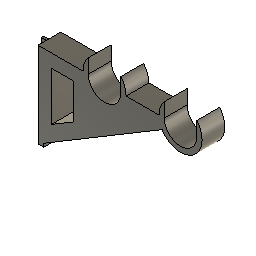
spool_cradle_bracket (Autodesk Fusion 360 design; units mm, degrees)
part number: 2026-09-02-15-42-23-246
Autodesk Fusion 360 part; units mm, degrees
sketch "Arm triangle" plane through (0, 0, 0) normal (0, 1, 0) x (1, 0, 0)
  line L0 (0, 0) -> (0, -90)
  line L1 (0, -90) -> (150, -90)
  line L2 (150, -90) -> (0, 0)
extrude "Arm triangle (1)" add sketch "Arm triangle" along normal mid plane 24
sketch "Hook plate" plane through (0, 0, 0) normal (0, 1, 0) x (1, 0, 0)
  line L0 (0, 0) -> (6, 0)
  line L1 (6, 0) -> (6, -90)
  line L2 (6, -90) -> (0, -90)
  line L3 (0, -90) -> (0, 0)
extrude "Hook plate (1)" add sketch "Hook plate" along normal mid plane 24
sketch "Lightening cutout" plane through (0, 0, 0) normal (0, 1, 0) x (1, 0, 0)
  line L0 (14, -24.7267) -> (14, -76)
  line L1 (14, -76) -> (37.3, -76)
  line L2 (37.3, -76) -> (37.3, -38.7067)
  line L3 (37.3, -38.7067) -> (14, -24.7267)
extrude "Lightening cutout (1)" cut sketch "Lightening cutout" along normal mid plane 34
sketch "Saddle boss x=70" plane through (0, 0, 0) normal (0, 1, 0) x (1, 0, 0)
  circle A0 centre (70, -90) radius 22.7
extrude "Saddle boss x=70 (1)" add sketch "Saddle boss x=70" along normal mid plane 24
sketch "Saddle boss x=150" plane through (0, 0, 0) normal (0, 1, 0) x (1, 0, 0)
  circle A0 centre (150, -90) radius 22.7
extrude "Saddle boss x=150 (1)" add sketch "Saddle boss x=150" along normal mid plane 24
sketch "Rod pocket x=70" plane through (0, 0, 0) normal (0, 1, 0) x (1, 0, 0)
  circle A0 centre (70, -90) radius 17.1
extrude "Rod pocket x=70 (1)" cut sketch "Rod pocket x=70" along normal mid plane 34
sketch "Drop-in opening x=70" plane through (0, 0, 0) normal (0, 1, 0) x (1, 0, 0)
  line L0 (52.9, -90) -> (87.1, -90)
  line L1 (87.1, -90) -> (87.1, -117.7)
  line L2 (87.1, -117.7) -> (52.9, -117.7)
  line L3 (52.9, -117.7) -> (52.9, -90)
extrude "Drop-in opening x=70 (1)" cut sketch "Drop-in opening x=70" along normal mid plane 34
sketch "Rod pocket x=150" plane through (0, 0, 0) normal (0, 1, 0) x (1, 0, 0)
  circle A0 centre (150, -90) radius 17.1
extrude "Rod pocket x=150 (1)" cut sketch "Rod pocket x=150" along normal mid plane 34
sketch "Drop-in opening x=150" plane through (0, 0, 0) normal (0, 1, 0) x (1, 0, 0)
  line L0 (132.9, -90) -> (167.1, -90)
  line L1 (167.1, -90) -> (167.1, -117.7)
  line L2 (167.1, -117.7) -> (132.9, -117.7)
  line L3 (132.9, -117.7) -> (132.9, -90)
extrude "Drop-in opening x=150 (1)" cut sketch "Drop-in opening x=150" along normal mid plane 34
sketch "Hook profiles" plane through (0, 0, 0) normal (0, 1, 0) x (1, 0, 0)
  line L0 (0, -88) -> (-7.3, -88)
  line L1 (-7.3, -88) -> (-7.3, -71)
  line L2 (-7.3, -71) -> (-2.8, -71)
  line L3 (-2.8, -71) -> (-2.8, -83)
  line L4 (-2.8, -83) -> (0, -83)
  line L5 (0, -83) -> (0, -88)
  line L6 (0, -62.6) -> (-7.3, -62.6)
  line L7 (-7.3, -62.6) -> (-7.3, -45.6)
  line L8 (-7.3, -45.6) -> (-2.8, -45.6)
  line L9 (-2.8, -45.6) -> (-2.8, -57.6)
  line L10 (-2.8, -57.6) -> (0, -57.6)
  line L11 (0, -57.6) -> (0, -62.6)
  line L12 (0, -37.2) -> (-7.3, -37.2)
  line L13 (-7.3, -37.2) -> (-7.3, -20.2)
  line L14 (-7.3, -20.2) -> (-2.8, -20.2)
  line L15 (-2.8, -20.2) -> (-2.8, -32.2)
  line L16 (-2.8, -32.2) -> (0, -32.2)
  line L17 (0, -32.2) -> (0, -37.2)
  line L18 (0, -11.8) -> (-7.3, -11.8)
  line L19 (-7.3, -11.8) -> (-7.3, 5.2)
  line L20 (-7.3, 5.2) -> (-2.8, 5.2)
  line L21 (-2.8, 5.2) -> (-2.8, -6.8)
  line L22 (-2.8, -6.8) -> (0, -6.8)
  line L23 (0, -6.8) -> (0, -11.8)
extrude "Hook column" add sketch "Hook profiles" along normal mid plane 2.4
named bodies: "spool_cradle_bracket"
